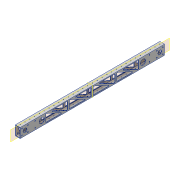
# Autodesk Inventor part: Support Pivs 25
Saved by Autodesk Inventor 2018 (Build 220112000, 112)
## iProperties
Created: 2018-01-08
Part Number: Support Pivs 25
Material: Aluminum 6061
Document SubType Name: Modeling
Designer: dsayers
Density: 2.7 g/cm^3
Appearance: Aluminum - Flat
Mass: 492.889 g
Surface Area: 1569.89 cm^2
Volume: 182.552 cm^3
Author: dsayers
Autodesk Inventor part; units mm, degrees
ref_plane "YZ Plane" through (0, 0, 0) normal (1, 0, 0) x (0, 1, 0)
ref_plane "XZ Plane" through (0, 0, 0) normal (0, 1, 0) x (-1, 0, 0)
ref_plane "XY Plane" through (0, 0, 0) normal (0, 0, 1) x (1, 0, 0)
sketch "Sketch1" plane through (0, 0, 0) normal (0, 0, 1) x (1, 0, 0)
  line L0 (0, 0) -> (25.4, 0)
  line L1 (25.4, 0) -> (25.4, 50.8)
  line L2 (25.4, 50.8) -> (0, 50.8)
  line L3 (0, 50.8) -> (0, 0)
  dimension "d0" = 25.4
  dimension "d1" = 50.8
  constraints: 8 end point, 2 parallel, 1 horizontal, 1 perpendicular
  measures "d0" distance of L1.end L2.end
  measures "d1" distance of L0.end L1.end
extrude "Extrusion1" add sketch "Sketch1" along normal blind 762
shell "Shell1" thickness 2.54 removed faces 2 at (8.4667, 33.8667, 0) at (8.4667, 33.8667, 762)
sketch "Sketch2" plane through (0, 50.8, 0) normal (0, 1, 0) x (1, 0, 0)
  line L0 (25.4, 0) -> (0, 0) projected
  line L1 (0, 0) -> (0, -762) projected
  point P0 (12.7, -12.7)
  point P1 (12.7, -38.1)
  point P2 (12.7, -63.5)
  point P3 (12.7, -88.9)
  point P4 (12.7, -114.3)
  point P5 (12.7, -139.7)
  point P6 (12.7, -165.1)
  point P7 (12.7, -190.5)
  point P8 (12.7, -215.9)
  point P9 (12.7, -241.3)
  point P10 (12.7, -266.7)
  point P11 (12.7, -292.1)
  point P12 (12.7, -317.5)
  point P13 (12.7, -342.9)
  point P14 (12.7, -368.3)
  point P15 (12.7, -393.7)
  point P16 (12.7, -419.1)
  point P17 (12.7, -444.5)
  point P18 (12.7, -469.9)
  point P19 (12.7, -495.3)
  point P20 (12.7, -520.7)
  point P21 (12.7, -546.1)
  point P22 (12.7, -571.5)
  point P23 (12.7, -596.9)
  point P24 (12.7, -622.3)
  point P25 (12.7, -647.7)
  point P26 (12.7, -673.1)
  point P27 (12.7, -698.5)
  point P28 (12.7, -723.9)
  point P29 (12.7, -749.3)
  point P30 (12.7, -774.7)
  point P31 (12.7, -800.1)
  point P32 (12.7, -825.5)
  point P33 (12.7, -850.9)
  point P34 (12.7, -876.3)
  point P35 (12.7, -901.7)
  point P36 (12.7, -927.1)
  dimension "d5" = 12.7
  dimension "d6" = 12.7
  dimension "d9" = 25.4
  constraints: 1 vertical, 36 other
  measures "d5" distance from line of L0 point (12.7, -12.7)
  measures "d6" distance from line of L1 point (12.7, -12.7)
  measures "d9" distance of point (12.7, -12.7) point (12.7, -38.1)
hole "Hole1" at (12.7, 50.8, 12.7) at (12.7, 50.8, 38.1) at (12.7, 50.8, 63.5) at (12.7, 50.8, 88.9) at (12.7, 50.8, 114.3) at (12.7, 50.8, 139.7) at (12.7, 50.8, 165.1) at (12.7, 50.8, 190.5) at (12.7, 50.8, 215.9) at (12.7, 50.8, 241.3) at (12.7, 50.8, 266.7) at (12.7, 50.8, 292.1) at (12.7, 50.8, 317.5) at (12.7, 50.8, 342.9) at (12.7, 50.8, 368.3) at (12.7, 50.8, 393.7) at (12.7, 50.8, 419.1) at (12.7, 50.8, 444.5) at (12.7, 50.8, 469.9) at (12.7, 50.8, 495.3) at (12.7, 50.8, 520.7) at (12.7, 50.8, 546.1) at (12.7, 50.8, 571.5) at (12.7, 50.8, 596.9) at (12.7, 50.8, 622.3) at (12.7, 50.8, 647.7) at (12.7, 50.8, 673.1) at (12.7, 50.8, 698.5) at (12.7, 50.8, 723.9) at (12.7, 50.8, 749.3) at (12.7, 50.8, 774.7) at (12.7, 50.8, 800.1) at (12.7, 50.8, 825.5) at (12.7, 50.8, 850.9) at (12.7, 50.8, 876.3) at (12.7, 50.8, 901.7) direction (0, -1, 0) diameter 2.54 depth 50.8 tip angle 118
sketch "Sketch6" plane through (25.4, 0, 0) normal (1, 0, 0) x (0, 0, -1)
  line L0 (0, 50.8) -> (-762, 50.8) projected
  line L1 (-762, 0) -> (-762, 50.8) projected
  line L2 (-742.0993, 34.925) -> (-731.1007, 34.925)
  line L3 (-731.1007, 34.925) -> (-725.6015, 25.4)
  line L4 (-725.6015, 25.4) -> (-731.1007, 15.875)
  line L5 (-731.1007, 15.875) -> (-742.0993, 15.875)
  line L6 (-742.0993, 15.875) -> (-747.5985, 25.4)
  line L7 (-747.5985, 25.4) -> (-742.0993, 34.925)
  point P0 (0, 0)
  point P1 (-736.6, 25.4)
  point P2 (-736.6, 25.4)
  dimension "d48" = 25.4
  dimension "d49" = 25.4
  dimension "d50" = 19.05
  constraints: 12 end point, 1 coincident, 1 parallel, 13 other
  measures "d48" distance from line of L0 point (-736.6, 25.4)
  measures "d49" distance from line of L1 point (-736.6, 25.4)
  measures "d50" distance between parallel lines of L5 L2
extrude "Extrusion2" cut sketch "Sketch6" against normal blind 25.4
sketch "Sketch8" plane through (25.4, 0, 0) normal (1, 0, 0) x (0, 0, -1)
  line L0 (-19.9007, 15.875) -> (-30.8993, 15.875)
  line L1 (-30.8993, 15.875) -> (-36.3985, 25.4)
  line L2 (-36.3985, 25.4) -> (-30.8993, 34.925)
  line L3 (-30.8993, 34.925) -> (-19.9007, 34.925)
  line L4 (-19.9007, 34.925) -> (-14.4015, 25.4)
  line L5 (-14.4015, 25.4) -> (-19.9007, 15.875)
  line L6 (0, 50.8) -> (-762, 50.8) projected
  line L7 (0, 0) -> (0, 50.8) projected
  point P0 (-25.4, 25.4)
  point P1 (-698.5, 50.8)
  dimension "d57" = 25.4
  dimension "d58" = 19.05
  dimension "d59" = 25.4
  constraints: 12 end point, 1 parallel, 13 other
  measures "d57" distance from line of L6 point (-25.4, 25.4)
  measures "d58" distance between parallel lines of L0 L3
  measures "d59" distance from line of L7 point (-25.4, 25.4)
extrude "Extrusion4" cut sketch "Sketch8" against normal blind 25.4
sketch "Sketch10" plane through (0, 0, 0) normal (-1, 0, 0) x (0, 0, 1)
  line L0 (0, 0) -> (762, 0) projected
  line L1 (0, 50.8) -> (762, 50.8) projected
  line L2 (0, 50.8) -> (0, 0) projected
  line L3 (19.9007, 34.925) -> (30.8993, 34.925) projected
  line L4 (30.8993, 15.875) -> (19.9007, 15.875) projected
  line L5 (0, 0) -> (762, 0) projected
  point P0 (9.525, 41.275)
  point P1 (41.275, 41.275)
  point P2 (79.375, 41.275)
  point P3 (79.375, 9.525)
  point P4 (41.275, 9.525)
  point P5 (9.525, 9.525)
  dimension "d66" = 9.525
  dimension "d67" = 9.525
  dimension "d68" = 9.525
  dimension "d69" = 9.525
  dimension "d72" = 31.75
  dimension "d74" = 9.525
  dimension "d75" = 38.1
  dimension "d76" = 38.1
  dimension "d77" = 9.525
  dimension "d78" = 9.525
  dimension "d79" = 9.525
  measures "d66" distance from line of L0 point (9.525, 9.525)
  measures "d67" distance from line of L1 point (9.525, 41.275)
  measures "d68" distance from line of L2 point (9.525, 41.275)
  measures "d69" distance from line of L2 point (9.525, 9.525)
  measures "d72" distance of point (9.525, 9.525) point (41.275, 9.525)
  measures "d74" distance from line of L5 point (41.275, 9.525)
  measures "d75" distance of point (41.275, 9.525) point (79.375, 9.525)
  measures "d76" distance of point (41.275, 41.275) point (79.375, 41.275)
  measures "d77" distance from line of L1 point (79.375, 41.275)
  measures "d78" distance from line of L1 point (41.275, 41.275)
  measures "d79" distance from line of L0 point (79.375, 9.525)
hole "Hole5" at (0, 41.275, 9.525) at (0, 41.275, 41.275) at (0, 41.275, 79.375) at (0, 9.525, 79.375) at (0, 9.525, 41.275) at (0, 9.525, 9.525) direction (1, 0, 0) diameter 5.1054 depth 25.4 tip angle 118 clearance for "Flat Head Machine Screw (82)" size "#10" standard "Ansi Unified Screw Threads"
ref_plane "Work Plane1" through (0, 0, 381) normal (0, 0, -1) x (-1, 0, 0)
mirror "Mirror1" about plane through (0, 0, 381) normal (0, 0, -1) of "Hole5"
sketch "Sketch11" plane through (0, 0, 0) normal (-1, 0, 0) x (0, 0, 1)
  circle A0 centre (114.3, 25.4) radius 14.2875
  line L0 (0, 50.8) -> (762, 50.8) projected
  circle A1 centre (647.7, 25.4) radius 14.2875
  line L1 (762, 50.8) -> (762, 0) projected
  line L2 (0, 50.8) -> (0, 0) projected
  line L3 (0, 0) -> (762, 0) projected
  dimension "d87" = 25.4
  dimension "d88" = 28.575
  dimension "d89" = 28.575
  dimension "d90" = 114.3
  dimension "d91" = 114.3
  dimension "d92" = 25.4
  constraints: 2 centre point
  measures "d87" distance from line of L0 A0.centre
  measures "d88" diameter of A0
  measures "d89" diameter of A1
  measures "d90" distance from line of L1 A1.centre
  measures "d91" distance from line of L2 A0.centre
  measures "d92" distance from line of L3 A1.centre
extrude "Extrusion6" cut sketch "Sketch11" against normal blind 25.4 contours A0 | A1
sketch "Sketch12" plane through (25.4, 0, 0) normal (1, 0, 0) x (0, 0, -1)
  line L0 (-139.7, 7.9375) -> (-139.7, 42.8625) construction
  line L1 (-136.4099, 7.9375) -> (-136.4099, 42.8625)
  line L2 (-142.9901, 42.8625) -> (-142.9901, 7.9375)
  arc A0 (-142.9901, 7.9375) -> (-136.4099, 7.9375) centre (-139.7, 7.9375) ccw
  arc A1 (-136.4099, 42.8625) -> (-142.9901, 42.8625) centre (-139.7, 42.8625) ccw
  line L3 (0, 0) -> (-762, 0) projected
  circle A2 centre (-114.3, 25.4) radius 14.2875 projected
  line L4 (-139.7, 7.9375) -> (-215.9, 42.8625) construction
  line L5 (-138.3292, 10.9284) -> (-214.5292, 45.8534)
  line L6 (-217.2708, 39.8716) -> (-141.0708, 4.9466)
  arc A3 (-141.0708, 4.9466) -> (-138.3292, 10.9284) centre (-139.7, 7.9375) ccw
  arc A4 (-214.5292, 45.8534) -> (-217.2708, 39.8716) centre (-215.9, 42.8625) ccw
  line L7 (-139.7, 42.8625) -> (-215.9, 42.8625) construction
  line L8 (-139.7, 39.5724) -> (-215.9, 39.5724)
  line L9 (-215.9, 46.1526) -> (-139.7, 46.1526)
  arc A5 (-139.7, 39.5724) -> (-139.7, 46.1526) centre (-139.7, 42.8625) ccw
  arc A6 (-215.9, 46.1526) -> (-215.9, 39.5724) centre (-215.9, 42.8625) ccw
  line L10 (-142.9901, 13.0646) -> (-142.9901, 39.5724)
  line L11 (-142.9901, 39.5724) -> (-200.8253, 39.5724)
  line L12 (-200.8253, 39.5724) -> (-142.9901, 13.0646)
  point P0 (-139.7, 25.4)
  point P1 (-177.8, 25.4)
  point P2 (-177.8, 42.8625)
  dimension "d100" = 25.4
  dimension "d101" = 34.925
  dimension "d102" = 25.4
  dimension "d103" = 76.2
  constraints: 30 end point, 12 point on circle, 12 tangent, 6 centre point, 6 point on line, 3 midpoint, 3 parallel, 1 collinear, 1 perpendicular, 1 vertical
  measures "d100" distance from line of L3 point (-139.7, 25.4)
  measures "d101" distance of L0.start L0.end
  measures "d102" distance from line of A2.centre L0
  measures "d103" distance of L0.end L4.end
extrude "Extrusion7" cut sketch "Sketch12" against normal blind 12.7 contours A3 L5 L2 L8 A5 L1 | A0 L2 L5 A3 | A5 L8 L2 A1 | L6 A6 L8 L5 L2 A0 | A1 L2 L8 L5 A4 L9 | A4 L5 L8 A6 | L5 L8 L2
sketch "Sketch13" plane through (25.4, 0, 0) normal (1, 0, 0) x (0, 0, -1)
  line L0 (-248.92, 42.8625) -> (-248.92, 7.9375) construction
  line L1 (-252.095, 42.8625) -> (-252.095, 7.9375)
  line L2 (-245.745, 7.9375) -> (-245.745, 42.8625)
  arc A0 (-245.745, 42.8625) -> (-252.095, 42.8625) centre (-248.92, 42.8625) ccw
  arc A1 (-252.095, 7.9375) -> (-245.745, 7.9375) centre (-248.92, 7.9375) ccw
  line L3 (0, 50.8) -> (-762, 50.8) projected
  line L4 (-248.92, 7.9375) -> (-172.72, 7.9375) construction
  line L5 (-248.92, 11.1125) -> (-172.72, 11.1125)
  line L6 (-172.72, 4.7625) -> (-248.92, 4.7625)
  arc A2 (-248.92, 11.1125) -> (-248.92, 4.7625) centre (-248.92, 7.9375) ccw
  arc A3 (-172.72, 4.7625) -> (-172.72, 11.1125) centre (-172.72, 7.9375) ccw
  line L7 (-172.72, 7.9375) -> (-248.92, 42.8625) construction
  line L8 (-171.3971, 10.8238) -> (-247.5971, 45.7488)
  line L9 (-250.2429, 39.9762) -> (-174.0429, 5.0512)
  arc A4 (-174.0429, 5.0512) -> (-171.3971, 10.8238) centre (-172.72, 7.9375) ccw
  arc A5 (-247.5971, 45.7488) -> (-250.2429, 39.9762) centre (-248.92, 42.8625) ccw
  line L10 (-245.745, 37.9147) -> (-245.745, 11.1125)
  line L11 (-245.745, 11.1125) -> (-187.2675, 11.1125)
  line L12 (-187.2675, 11.1125) -> (-245.745, 37.9147)
  arc A6 (-141.0708, 4.9466) -> (-136.4099, 7.9375) centre (-139.7, 7.9375) ccw projected
  line L13 (-245.745, 37.9147) -> (-245.745, 11.1125)
  line L14 (-245.745, 11.1125) -> (-187.2675, 11.1125)
  line L15 (-187.2675, 11.1125) -> (-245.745, 37.9147)
  line L16 (-187.2675, 11.1125) -> (-245.745, 37.9147)
  line L17 (-245.745, 37.9147) -> (-245.745, 11.5858)
  line L18 (-245.745, 37.9147) -> (-245.745, 11.5858)
  line L19 (-245.745, 11.1125) -> (-187.2675, 11.1125)
  line L20 (-187.2675, 11.1125) -> (-245.745, 37.9147)
  line L21 (-245.745, 37.9147) -> (-245.745, 11.1125)
  point P0 (0, 0)
  point P1 (-248.92, 25.4)
  point P2 (-210.82, 7.9375)
  point P3 (-210.82, 25.4)
  dimension "d106" = 6.35
  dimension "d107" = 25.4
  dimension "d108" = 34.925
  dimension "d109" = 76.2
  dimension "d110" = 33.02
  constraints: 48 end point, 12 point on circle, 12 tangent, 7 point on line, 6 centre point, 6 collinear, 3 midpoint, 3 parallel, 3 perpendicular, 2 vertical
  measures "d106" distance between parallel lines of L1 L2
  measures "d107" distance from line of L3 point (-248.92, 25.4)
  measures "d108" distance of L0.start L0.end
  measures "d109" distance of L0.end L4.end
  measures "d110" distance of A6.centre L4.end
extrude "Extrusion8" cut sketch "Sketch13" against normal blind 12.7
pattern_linear "Rectangular Pattern1" count 4 spacing 125.095 along (0, 0, 1) of "Extrusion8", "Extrusion7"
ref_plane "Work Plane2" through (12.7, 0, 0) normal (1, 0, 0) x (0, 0, -1)
mirror "Mirror2" about plane through (12.7, 0, 0) normal (1, 0, 0) of "Extrusion8", "Extrusion7", "Rectangular Pattern1"
equation "\"d68\" = d67"
equation "\"d69\" = d68"
equation "\"d72\" = 2 * d70"
equation "\"d74\" = d66"
equation "\"d76\" = d75"
equation "\"d77\" = d74"
equation "\"d78\" = d77"
equation "\"d79\" = d77"
equation "\"d89\" = d88"
equation "\"d91\" = d90"
equation "\"d70\" = 15.875"
body "Solid1"
